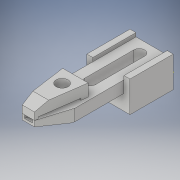
# Autodesk Inventor part: clamp_v2_1inch_slot_v1
Saved by Autodesk Inventor 2017 (Build 210142000, 142)
## iProperties
Created: 2016-07-15
Part Number: clamp_v2_1inch_slot_v1
Material: Generic
Document SubType Name: Modeling
Designer: Gergo_PC
Density: 1 g/cm^3
Appearance: Default
Author: Gergo_PC
Autodesk Inventor part; units mm, degrees
ref_plane "YZ Plane" through (0, 0, 0) normal (1, 0, 0) x (0, 1, 0)
sketch "Sketch1" plane through (0, 0, 0) normal (0, 1, 0) x (-1, 0, 0)
  line L0 (0, 0) -> (12.8347, 0)
  line L1 (12.8347, 0) -> (12.8347, 37.9512)
  line L2 (8.9346, 50.7079) -> (3.9001, 50.7079)
  line L3 (0, 37.9512) -> (0, 0)
  line L4 (8.9346, 50.7079) -> (12.8347, 37.9512)
  line L5 (3.9001, 50.7079) -> (0, 37.9512)
  line L6 (8.4266, 50.7079) -> (8.9346, 50.7079) construction
  circle A0 centre (6.4174, 36.83) radius 1.7272
  arc A1 (4.1695, 5.08) -> (8.6653, 5.08) centre (6.4174, 5.08) ccw
  arc A2 (8.6653, 25.4) -> (4.1695, 25.4) centre (6.4174, 25.4) ccw
  line L7 (8.6653, 25.4) -> (8.6653, 5.08)
  line L8 (4.1695, 25.4) -> (4.1695, 5.08)
  dimension "d10" = 3.4544
  dimension "d12" = 4.4958
  dimension "d13" = 5.08
  dimension "d14" = 4.4958
  dimension "d15" = 25.4
  dimension "d52" = 6.4173
  dimension "d53" = 12.8347
  dimension "d57" = 163
  dimension "d58" = 163
  dimension "d59" = 5.0345
  dimension "d60" = 6.4173
  dimension "d61" = 6.4173
  constraints: 18 end point, 4 point on circle, 3 centre point, 3 tangent, 2 horizontal, 2 parallel, 1 perpendicular, 1 point on line
  measures "d10" diameter of A0
  measures "d12" diameter of A1
  measures "d13" distance from line of L0 A1.centre
  measures "d14" diameter of A2
  measures "d15" distance from line of L0 A2.centre
  measures "d52" distance from line of L1 A0.centre
  measures "d53" distance between parallel lines of L3 L1
  measures "d57" angle of L1 L4
  measures "d58" angle of L3 L5
  measures "d59" distance of L2.start L2.end
  measures "d60" distance from line of L1 A1.centre
  measures "d61" distance from line of L1 A2.centre
ref_plane "Work Plane2" through (0, 4.826, 0) normal (0, 1, 0) x (1, 0, 0)
extrude "Extrusion3" add sketch "Sketch1" along normal blind 4.826
chamfer "Chamfer2" distance 2.54 distance2 11.43 1 edges at (-6.4174, 0, 50.7079) measured on face at (-7.2564, 1.6087, 50.7079)
sketch "Sketch12" plane through (0, 4.826, 0) normal (0, 1, 0) x (1, 0, 0)
  line L0 (-3.9001, -50.7079) -> (-8.9346, -50.7079) projected
  line L1 (-4.6964, -50.7079) -> (-5.6147, -47.0249)
  line L2 (-5.6147, -47.0249) -> (-7.1387, -47.0249)
  line L3 (-7.1387, -47.0249) -> (-8.057, -50.7079)
  line L4 (-8.9346, -50.7079) -> (-3.9001, -50.7079) projected
  point P0 (0, 0)
  dimension "d67" = 1.524
  dimension "d68" = 104
  dimension "d69" = 104
  dimension "d70" = 3.683
  dimension "d71" = 0.8776
  dimension "d72" = 5.0345
  constraints: 6 end point, 2 parallel, 2 point on line
  measures "d67" distance of L1.end L2.end
  measures "d68" angle of L3 L2
  measures "d69" angle of L1 L2
  measures "d70" distance between parallel lines of L0 L2
  measures "d71" distance of L0.end L3.end
  measures "d72" distance of L0.start L0.end
extrude "Extrusion4" cut sketch "Sketch12" against normal blind 1.27
sketch "Sketch13" plane through (0, 4.826, 0) normal (0, 1, 0) x (1, 0, 0)
  line L0 (-12.8347, -37.9512) -> (-8.9346, -50.7079) projected
  line L1 (-8.9346, -50.7079) -> (-3.9054, -50.7079)
  line L2 (-3.9054, -50.7079) -> (-1.1849, -31.3501)
  line L3 (-1.1849, -31.3501) -> (-11.6552, -31.3501)
  line L4 (-11.6552, -31.3501) -> (-8.9346, -50.7079)
  circle A0 centre (-6.4174, -36.83) radius 2.4638
  circle A1 centre (-6.4174, -36.83) radius 1.7272 projected
  line L5 (-3.9001, -50.7079) -> (-8.9346, -50.7079) projected
  point P0 (0, 0)
  dimension "d75" = 4.9276
  dimension "d76" = 5.0292
  dimension "d86" = 98
  dimension "d88" = 98
  constraints: 8 end point, 1 centre point, 1 concentric, 1 horizontal, 1 parallel
  measures "d75" diameter of A0
  measures "d76" distance of L0.end L1.end
  measures "d86" angle of L1 L4
  measures "d88" angle of L1 L2
extrude "Extrusion5" add sketch "Sketch13" along normal blind 5.08 contours L4 L3 L2 L1
split body "Split1" result two bodies by plane through (0, 4.826, 0) normal (0, 1, 0) first body at (-6.5181, 9.406, 46.8972)
chamfer "Chamfer3" distance 5.08 distance2 2.032 1 edges at (-6.42, 9.906, 50.7079) measured on face at (-6.5181, 9.906, 46.8972)
sketch "Sketch14" plane through (0, 4.826, 0) normal (0, -1, 0) x (1, 0, 0)
  line L0 (-3.7137, 49.3439) -> (-9.1263, 49.3439)
  line L1 (-9.1263, 49.3439) -> (-11.2887, 33.9578)
  line L2 (-11.2887, 33.9578) -> (-1.5513, 33.9578)
  line L3 (-1.5513, 33.9578) -> (-3.7137, 49.3439)
  line L4 (-1.1849, 31.3501) -> (-3.9054, 50.7079) projected
  line L5 (-8.9346, 50.7079) -> (-11.6552, 31.3501) projected
  point P0 (0, 0)
  constraints: 8 end point, 2 collinear, 1 equal length, 1 horizontal, 1 parallel, 1 other
extrude "Extrusion6" cut sketch "Sketch14" against normal blind 0.762 bodies 2
sketch "Sketch15" plane through (0, 0, 0) normal (0, -1, 0) x (1, 0, 0)
  line L0 (-15.3074, 17.78) -> (2.4726, 17.78)
  line L1 (2.4726, 17.78) -> (2.4726, 0)
  line L2 (2.4726, 0) -> (-15.3074, 0)
  line L3 (-15.3074, 0) -> (-15.3074, 17.78)
  line L4 (0, 0) -> (-12.8347, 0) projected
  circle A0 centre (-6.4174, 8.89) radius 2.2479
  point P0 (-6.4174, 0)
  dimension "d89" = 17.78
  dimension "d90" = 17.78
  dimension "d91" = 4.4958
  dimension "d92" = 8.89
  dimension "d93" = 8.89
  constraints: 8 end point, 2 midpoint, 2 parallel, 1 centre point, 1 horizontal, 1 perpendicular
  measures "d89" distance of L1.end L2.end
  measures "d90" distance of L0.end L1.end
  measures "d91" diameter of A0
  measures "d92" distance from line of L3 A0.centre
  measures "d93" distance from line of L0 A0.centre
extrude "Extrusion7" add sketch "Sketch15" along normal blind 6.35 bodies 3
sketch "Sketch16" plane through (0, 4.826, 0) normal (0, 0, -1) x (-1, 0, 0)
  line L0 (-2.4726, -4.826) -> (0, -4.826) projected
  line L1 (12.8378, -4.826) -> (0, -4.826)
  constraints: 2 end point, 1 collinear
ref_plane "Work Plane3" through (-15.3074, 0, 0) normal (0, 1, 0) x (1, 0, 0)
split body "Split2" result two bodies by plane through (-15.3074, 0, 0) normal (0, 1, 0) bodies 3 first body at (-11.4449, 4.326, 21.1171)
sketch "Sketch17" plane through (0, 0, 0) normal (0, 1, 0) x (1, 0, 0)
  line L0 (0, -37.9512) -> (0, 0) projected
  line L1 (0, -17.78) -> (2.4726, -17.78)
  line L2 (2.4726, -17.78) -> (2.4726, 0)
  line L3 (2.4726, 0) -> (0, 0)
  line L4 (0, 0) -> (0, -17.78)
  line L5 (2.4726, 0) -> (-15.3074, 0) projected
  line L6 (-12.8347, 0) -> (-12.8347, -37.9512) projected
  line L7 (-15.3074, 0) -> (-12.8347, 0)
  line L8 (-12.8347, 0) -> (-12.8347, -17.78)
  line L9 (-12.8347, -17.78) -> (-15.3074, -17.78)
  line L10 (-15.3074, -17.78) -> (-15.3074, 0)
  line L11 (2.4726, -17.78) -> (2.4726, 0) projected
  line L12 (-15.3074, -17.78) -> (2.4726, -17.78) projected
  point P0 (2.4726, -8.89)
  point P1 (-14.071, -17.78)
  constraints: 16 end point, 4 parallel, 4 point on line, 3 midpoint, 2 horizontal, 2 perpendicular
extrude "Extrusion8" add sketch "Sketch17" along normal blind 6.35 contours L0 L3 L2 L1 | L9 L10 L5 L6 bodies 5
equation "\"d52\" = 0.5 * d53"
equation "\"d60\" = 0.5 * d53"
equation "\"d61\" = 0.5 * d53"
equation "\"d71\" = -0.25 * d67 + 0.25 * d72"
equation "\"d23\" = 0.5 * d24"
equation "\"d24\" = 12.7"
body "Solid2"
body "Solid4"
body "Solid5"
